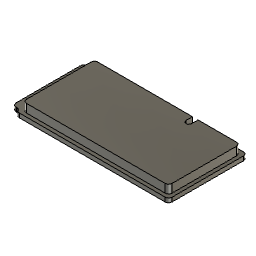
Waterproofing case - TPU lid (Autodesk Fusion 360 design; units mm, degrees)
Autodesk Fusion 360 part; units mm, degrees
sketch "Sketch1" plane through (0, 0, 0) normal (0, 0, 1) x (1, 0, 0)
  line L0 (0, 0) -> (104, 0)
  line L1 (104, 0) -> (104, 51)
  line L2 (104, 51) -> (0, 51)
  line L3 (0, 51) -> (0, 0)
  dimension "d1" = 104
  dimension "d2" = 51
  constraint horizontal L0
  constraint vertical L1
  constraint horizontal L2
  constraint vertical L3
  constraint coincident L0.start L3.end
  measures "d1" distance of L0.start L0.end
  measures "d2" distance of L0.start L2.end
extrude "Extrude1" add sketch "Sketch1" along normal blind 4
fillet "Fillet1" radius 2.5 4 edges at (104, 0, 2) (0, 0, 2) (104, 51, 2) (0, 51, 2)
sketch "Sketch2" plane through (0, 0, 4) normal (0, 0, 1) x (-1, 0, 0)
  arc A0 (-2.5, -51) -> (0, -48.5) centre (-2.5, -48.5) ccw
  line L0 (0, -48.5) -> (0, -2.5)
  arc A1 (0, -2.5) -> (-2.5, 0) centre (-2.5, -2.5) ccw
  line L1 (-2.5, 0) -> (-101.5, 0)
  arc A2 (-101.5, 0) -> (-104, -2.5) centre (-101.5, -2.5) ccw
  line L2 (-104, -2.5) -> (-104, -48.5)
  arc A3 (-104, -48.5) -> (-101.5, -51) centre (-101.5, -48.5) ccw
  line L3 (-101.5, -51) -> (-2.5, -51)
sketch "Sketch3" plane through (0, 0, 4) normal (0, 0, 1) x (-1, 0, 0)
  line L0 (2, -53) -> (-106, -53)
  line L1 (-106, -53) -> (-106, 2)
  line L2 (-106, 2) -> (2, 2)
  line L3 (2, 2) -> (2, -53)
  line L4 (-2.5, 0) -> (-101.5, 0)
  line L5 (-104, -2.5) -> (-104, -48.5)
  line L6 (0, -48.5) -> (0, -2.5)
  line L7 (-101.5, -51) -> (-2.5, -51)
  dimension "d7" = 2
  dimension "d8" = 2
  dimension "d9" = 2
  dimension "d10" = 2
  constraint horizontal L0
  constraint vertical L1
  constraint horizontal L2
  constraint vertical L3
  measures "d7" distance of L2 L4
  measures "d8" distance of L1 L5
  measures "d9" distance of L3 L6
  measures "d10" distance of L0 L7
sketch "Sketch6" plane through (0, 0, 0) normal (0, 0, 1) x (1, 0, 0)
  line L0 (-2.5, -2.5) -> (106.5, -2.5)
  line L1 (106.5, -2.5) -> (106.5, 53.5)
  line L2 (106.5, 53.5) -> (-2.5, 53.5)
  line L3 (-2.5, 53.5) -> (-2.5, -2.5)
  line L4 (2.5, 0) -> (101.5, 0)
  line L5 (104, 2.5) -> (104, 48.5)
  line L6 (101.5, 51) -> (2.5, 51)
  line L7 (0, 48.5) -> (0, 2.5)
  dimension "d15" = 2.5
  dimension "d16" = 2.5
  dimension "d17" = 2.5
  dimension "d18" = 2.5
  constraint horizontal L0
  constraint vertical L1
  constraint horizontal L2
  constraint vertical L3
  measures "d15" distance of L0 L4
  measures "d16" distance of L1 L5
  measures "d17" distance of L2 L6
  measures "d18" distance of L3 L7
extrude "Extrude3" add sketch "Sketch6" against normal blind 3
fillet "Fillet3" radius 2.5 4 edges at (-2.5, 53.5, -1.5) (106.5, 53.5, -1.5) (106.5, -2.5, -1.5) (-2.5, -2.5, -1.5)
sketch "Sketch7" plane through (0, 0, 4) normal (0, 0, 1) x (-1, 0, 0)
  circle A0 centre (-34, -46.5) radius 2.5
  line L0 (-104, -2.5) -> (-104, -48.5)
  line L1 (-101.5, -51) -> (-2.5, -51)
  line L2 (-36.5, -46.5) -> (-36.5, -51)
  line L3 (-31.5, -46.5) -> (-31.5, -51)
  dimension "d23" = 5
  dimension "d24" = 70
  dimension "d25" = 4.5
  constraint coincident A0 L2.start
  constraint coincident L1 L2.end
  constraint tangent A0 L2
  constraint perpendicular L1 L2
  constraint coincident A0 L3.start
  constraint coincident L1 L3.end
  constraint tangent A0 L3
  constraint perpendicular L1 L3
  measures "d23" diameter of A0
  measures "d24" distance of A0.centre L0
  measures "d25" distance of A0.centre L1
extrude "Extrude4" cut sketch "Sketch7" against normal blind 11
sketch "Sketch8" plane through (0, 0, -3) normal (0, 0, -1) x (1, 0, 0)
  line L0 (36.5, -51) -> (31.5, -51)
  line L1 (31.5, -51) -> (31.5, -46.5)
  arc A0 (36.5, -46.5) -> (31.5, -46.5) centre (34, -46.5) ccw
  line L2 (36.5, -46.5) -> (36.5, -51)
  arc A1 (0, 2.5) -> (-2.5, 0) centre (0, 0) ccw
  line L3 (-2.5, 0) -> (-2.5, -51)
  arc A2 (-2.5, -51) -> (0, -53.5) centre (0, -51) ccw
  line L4 (0, -53.5) -> (104, -53.5)
  arc A3 (104, -53.5) -> (106.5, -51) centre (104, -51) ccw
  line L5 (106.5, -51) -> (106.5, 0)
  arc A4 (106.5, 0) -> (104, 2.5) centre (104, 0) ccw
  line L6 (104, 2.5) -> (0, 2.5)
  line L7 (31.5, -51) -> (31.5, -53.5)
  line L8 (36.5, -51) -> (36.5, -53.5)
  constraint coincident L0.end L1.start
  constraint coincident L4 L7.end
  constraint perpendicular L4 L7
  constraint coincident L0.start L2.end
  constraint coincident L4 L8.end
  constraint perpendicular L4 L8
extrude "Extrude5" cut sketch "Sketch8" against normal blind 4 contours L0 L4 L7 L8
sketch "Sketch9" plane through (0, 0, 4) normal (0, 0, 1) x (-1, 0, 0)
sketch "Sketch10" plane through (0, 0, 4) normal (0, 0, 1) x (-1, 0, 0)
sketch "Sketch11" plane through (0, 0, -3) normal (0, 0, -1) x (1, 0, 0)
  line L0 (36.5, -46.5) -> (36.5, -53.5)
  line L1 (36.5, -53.5) -> (104, -53.5)
  arc A0 (104, -53.5) -> (106.5, -51) centre (104, -51) ccw
  line L2 (106.5, -51) -> (106.5, 0)
  arc A1 (106.5, 0) -> (104, 2.5) centre (104, 0) ccw
  line L3 (104, 2.5) -> (0, 2.5)
  arc A2 (0, 2.5) -> (-2.5, 0) centre (0, 0) ccw
  line L4 (-2.5, 0) -> (-2.5, -51)
  arc A3 (-2.5, -51) -> (0, -53.5) centre (0, -51) ccw
  line L5 (0, -53.5) -> (31.5, -53.5)
  line L6 (31.5, -53.5) -> (31.5, -46.5)
  arc A4 (36.5, -46.5) -> (31.5, -46.5) centre (34, -46.5) ccw
  line L7 (70, -53.5) -> (74, -53.5)
  line L8 (74, -53.5) -> (74, -46.5)
  line L9 (74, -46.5) -> (70, -46.5)
  line L10 (70, -46.5) -> (70, -53.5)
  circle A5 centre (72, -46.5) radius 2
  dimension "d30" = 32.5
  dimension "d31" = 4
  dimension "d32" = 7
  constraint horizontal L7
  constraint vertical L8
  constraint horizontal L9
  constraint vertical L10
  constraint coincident L1 L7.start
  constraint midpoint L9 A5.centre
  constraint coincident L8.end A5
  measures "d30" distance of L2 L8
  measures "d31" distance of L8 L10
  measures "d32" distance of L7.start L9.end
extrude "Extrude6" cut sketch "Sketch11" against normal blind 9 contours L1 L7 L8 L10 A5 | L9 A5 | L9 A5
extrude "Extrude7" add sketch "Sketch7" against normal blind 7
extrude "Extrude8" add sketch "Sketch8" against normal blind 3 contours L0 L4 L7 L8
extrude "Extrude9" add sketch "Sketch2" along normal blind 2
extrude "Extrude10" cut 1 faces at (72.6667, 48, 4) along direction (0, 0, 1) blind 9
extrude "Extrude11" add 1 faces at (-2.5, 34, -1) along direction (-1, 0, 0) blind 5
fillet "Fillet4" radius 2.5 4 edges at (-7.5, 51, -1.5) (-2.5, 51, -1.5) (-2.5, 0, -1.5) (-7.5, 0, -1.5)
sketch "Sketch12" plane through (0, 0, 0) normal (0, 1, 0) x (1, 0, 0)
extrude "Extrude12" [suppressed]
extrude "Extrude2" [suppressed]
fillet "Fillet2" [suppressed]
sketch "Sketch4" plane through (0, 0, 0) normal (0, 0, 1) x (1, 0, 0)
sketch "Sketch5" plane through (0, 0, 0) normal (0, 0, 1) x (1, 0, 0)
